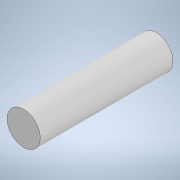
# Autodesk Inventor part: Connector
Saved by Autodesk Inventor 2022 (Build 260153000, 153)
## iProperties
Created: 2022-02-07
Part Number: Connector
Material: Generic
Document SubType Name: Modeling
Designer: mogje
Density: 1 g/cm^3
Appearance: Default
Author: mogje
Autodesk Inventor part; units mm, degrees
ref_plane "YZ Plane" through (0, 0, 0) normal (1, 0, 0) x (0, 1, 0)
ref_plane "XZ Plane" through (0, 0, 0) normal (0, 1, 0) x (-1, 0, 0)
ref_plane "XY Plane" through (0, 0, 0) normal (0, 0, 1) x (1, 0, 0)
sketch "Sketch1" plane through (0, 0, 0) normal (0, 1, 0) x (-1, 0, 0)
  line L0 (0, 0) -> (0, 1.524)
  line L1 (0, 1.524) -> (0.381, 1.524)
  line L2 (0.381, 1.524) -> (0.381, 0)
  line L3 (0, 0) -> (0, -1.524)
  line L4 (0, -1.524) -> (0.381, -1.524)
  line L5 (0.381, -1.524) -> (0.381, 0)
  dimension "d0" = 1.524
  dimension "d1" = 0.381
  constraints: 12 end point, 1 parallel, 1 perpendicular, 1 vertical
  measures "d0" distance of L0.start L0.end
  measures "d1" distance of L0.end L1.end
revolve "Revolution1" add sketch "Sketch1" angle 360 about axis through (0, 0, 0) along (0, 0, -1)
body "Solid1"
